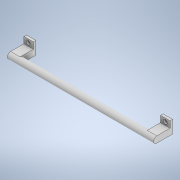
# Autodesk Inventor part: Model1_P3
Saved by Autodesk Inventor 2021 (Build 250183000, 183)
## iProperties
Created: 2021-02-04
Part Number: Model1_P3
Material: Generic
Document SubType Name: Modeling
Designer: nevkd
Density: 1 g/cm^3
Appearance: Default
Author: nevkd
Autodesk Inventor part; units mm, degrees
ref_plane "YZ Plane" through (0, 0, 0) normal (1, 0, 0) x (0, 1, 0)
ref_plane "XZ Plane" through (0, 0, 0) normal (0, 1, 0) x (-1, 0, 0)
ref_plane "XY Plane" through (0, 0, 0) normal (0, 0, 1) x (1, 0, 0)
sketch "Sketch1" plane through (0, 0, 0) normal (1, 0, 0) x (0, 1, 0)
  circle A0 centre (0, 0) radius 5
  dimension "d0" = 10
  constraints: 1 centre point, 1 coincident
  measures "d0" diameter of A0
extrude "Extrusion1" add sketch "Sketch1" along normal blind 200
sketch "Sketch2" plane through (200, 0, 0) normal (1, 0, 0) x (0, 0, -1)
  circle A0 centre (0, 0) radius 5 projected
  arc A1 (0, 5) -> (0, -5) centre (0, 0) ccw
  line L0 (0, 5) -> (0, -5)
  constraints: 4 point on circle, 2 end point, 1 centre point, 1 concentric, 1 vertical
extrude "Extrusion2" add sketch "Sketch2" along normal blind 15 contours L0 A0 picked at (-0.7745, -1.4758)
sketch "Sketch3" plane through (200, -5, 0) normal (0, 0, -1) x (-1, 0, 0)
  point P0 (200, 5)
sketch "Sketch4" plane through (200, -5, 0) normal (0, 0, -1) x (-1, 0, 0)
  line L0 (-15, 10) -> (-15, 0) projected
  line L1 (0, 10) -> (0, 0) projected
  line L2 (-15, 10) -> (0, 10)
  line L3 (0, 10) -> (0, 0)
  line L4 (0, 0) -> (-15, 0)
  line L5 (-15, 0) -> (-15, 10)
  point P0 (200, 5)
  constraints: 8 end point, 2 parallel, 1 horizontal, 1 perpendicular
extrude "Extrusion3" add sketch "Sketch4" along normal blind 25
sketch "Sketch7" plane through (200, 5, 0) normal (0, 1, 0) x (1, 0, 0)
  line L0 (0, 0) -> (0, 25) projected
  line L1 (15, 25) -> (0, 25)
  line L2 (0, 25) -> (0, 21)
  line L3 (0, 21) -> (15, 21)
  line L4 (15, 21) -> (15, 25)
  point P0 (-200, 0)
  dimension "d12" = 4
  constraints: 8 end point, 2 parallel, 1 horizontal, 1 perpendicular, 1 point on line
  measures "d12" distance of L3.end L1.start
extrude "Extrusion6" add sketch "Sketch7" along normal blind 10
sketch "Sketch8" plane through (0, 0, 0) normal (-1, 0, 0) x (0, 0, 1)
  circle A0 centre (0, 0) radius 5 projected
  line L0 (0, 5) -> (0, -5)
  arc A1 (0, -5) -> (0, 5) centre (0, 0) ccw
  dimension "d15" = 10
  constraints: 4 point on circle, 2 end point, 1 centre point, 1 concentric, 1 vertical
  measures "d15" distance of L0.start L0.end
extrude "Extrusion7" add sketch "Sketch8" along normal blind 15 contours A0 L0 picked at (1.0391, 1.3031)
sketch "Sketch9" plane through (0, -5, 0) normal (0, 0, -1) x (-1, 0, 0)
  line L0 (0, 10) -> (15, 10) projected
  line L1 (0, 10) -> (0, 0) projected
  line L2 (15, 10) -> (0, 10)
  line L3 (0, 10) -> (0, 0)
  line L4 (0, 0) -> (15, 0)
  line L5 (15, 0) -> (15, 10)
  point P0 (0, 5)
  constraints: 8 end point, 2 parallel, 1 horizontal, 1 perpendicular
extrude "Extrusion8" add sketch "Sketch9" along normal blind 25
sketch "Sketch10" plane through (-15, 5, 0) normal (0, 1, 0) x (1, 0, 0)
  line L0 (0, 25) -> (15, 25) projected
  line L1 (0, 0) -> (0, 25) projected
  line L2 (15, 25) -> (0, 25)
  line L3 (0, 25) -> (0, 21)
  line L4 (0, 21) -> (15, 21)
  line L5 (15, 21) -> (15, 25)
  point P0 (15, 0)
  dimension "d20" = 4
  constraints: 8 end point, 2 parallel, 1 horizontal, 1 perpendicular, 1 point on line
  measures "d20" distance of L4.end L0.end
extrude "Extrusion9" add sketch "Sketch10" along normal blind 10
sketch "Sketch11" plane through (-15, 5, -21) normal (0, 0, 1) x (1, 0, 0)
  point P0 (15, -5)
sketch "Sketch12" plane through (200, 5, -21) normal (0, 0, 1) x (1, 0, 0)
  circle A0 centre (7.5, 5) radius 3.265
  line L0 (0, 10) -> (15, 10) projected
  line L1 (0, 0) -> (0, 10) projected
  point P0 (-200, -5)
  dimension "d23" = 6.53
  dimension "d24" = 5
  dimension "d25" = 7.5
  constraints: 1 centre point
  measures "d23" diameter of A0
  measures "d24" distance from line of L0 A0.centre
  measures "d25" distance from line of L1 A0.centre
extrude "Extrusion10" cut sketch "Sketch12" against normal blind 2.8
sketch "Sketch13" plane through (207.5, 10, -23.8) normal (0, 0, 1) x (1, 0, 0)
  circle A0 centre (0, 0) radius 3.265 projected
  point P0 (-207.5, -10)
  constraints: 1 coincident
hole "Hole1" at (207.5, 10, -23.8) direction (0, 0, -1) diameter 4 end through all
sketch "Sketch14" plane through (-15, 5, -21) normal (0, 0, 1) x (1, 0, 0)
  circle A0 centre (6.6, 5) radius 3.265
  line L0 (0, 10) -> (15, 10) projected
  line L1 (215, 0) -> (215, 10) projected
  point P0 (15, -5)
  dimension "d35" = 6.53
  dimension "d36" = 5
  dimension "d37" = 208.4
  constraints: 1 centre point
  measures "d35" diameter of A0
  measures "d36" distance from line of L0 A0.centre
  measures "d37" distance from line of L1 A0.centre
extrude "Extrusion11" cut sketch "Sketch14" against normal blind 2.8
sketch "Sketch15" plane through (-8.4, 10, -23.8) normal (0, 0, 1) x (1, 0, 0)
  circle A0 centre (0, 0) radius 3.265 projected
  point P0 (8.4, -10)
  constraints: 1 coincident
hole "Hole2" at (-8.4, 10, -23.8) direction (0, 0, -1) diameter 4 end through all
body "Solid1"
